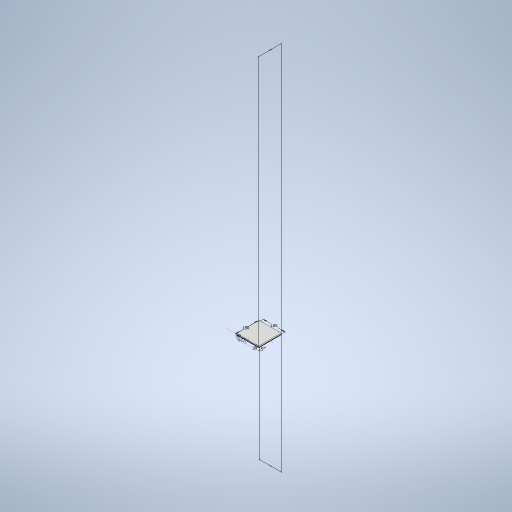
# Autodesk Inventor part: Coperchio
Saved by Autodesk Inventor 2024.2 (Build 282272000, 272)
## iProperties
Created: 2025-05-23
Part Number: Coperchio
Material: Generico
Document SubType Name: Modeling
Designer: zagom
Density: 1 g/cm^3
Appearance: Default
Author: zagom
Autodesk Inventor part; units mm, degrees
ref_plane "YZ Plane" through (0, 0, 0) normal (1, 0, 0) x (0, 1, 0)
ref_plane "XZ Plane" through (0, 0, 0) normal (0, 1, 0) x (-1, 0, 0)
ref_plane "XY Plane" through (0, 0, 0) normal (0, 0, 1) x (1, 0, 0)
sketch "Schizzo1" plane through (0, 0, 0) normal (0, 1, 0) x (-1, 0, 0)
  line L0 (-92.5, 95) -> (92.5, 95)
  line L1 (92.5, 95) -> (92.5, -95)
  line L2 (92.5, -95) -> (-92.5, -95)
  line L3 (-92.5, -95) -> (-92.5, 95)
  line L4 (-92.5, 95) -> (92.5, -95) construction
  line L5 (92.5, 95) -> (-92.5, -95) construction
  line L6 (118.5475, 95) -> (118.5475, 92.5) construction
  line L7 (103.3404, 0) -> (-125.0969, 0) construction
  line L8 (-92.5, 105.425) -> (-72.5, 105.425) construction
  line L9 (-72.5, 105.425) -> (-72.5, 79.9214) construction
  line L10 (-107.0445, 95) -> (-107.0445, 90) construction
  line L11 (-107.0445, 90) -> (178.9219, 90) construction
  line L12 (92.5, 110.0374) -> (62.5, 110.0374) construction
  line L13 (62.5, 110.0374) -> (62.5, 64.1892) construction
  line L14 (62.5, 124.2105) -> (-5, 124.2105) construction
  line L15 (-5, 124.2105) -> (-72.5, 124.2105) construction
  line L16 (-5, 124.2105) -> (-5, 64.1892) construction
  point P0 (0, 0)
  point P1 (62.5, 90)
  point P2 (-72.5, 90)
  point P3 (-5, 90)
  dimension "d0" = 185
  dimension "d1" = 190
  dimension "d39" = 20
  dimension "d40" = 5
  dimension "d41" = 30
  dimension "d57" = 67.5
  constraints: 34 end point, 7 point on line, 6 horizontal, 5 perpendicular, 2 midpoint, 2 parallel, 2 vertical
  measures "d0" distance of L1.end L2.end
  measures "d1" distance of L0.end L1.end
  measures "d39" distance of L8.start L8.end
  measures "d40" distance of L10.start L10.end
  measures "d41" distance of L12.start L12.end
  measures "d57" distance of L14.start L14.end
extrude "Estrusione1" add sketch "Schizzo1" along normal blind 10
ref_plane "Piano di lavoro1" through (-103.3404, 0, 0) normal (0, 0, 1) x (1, 0, 0)
hole "Foro5" at (-62.5, 0, 90) at (72.5, 0, 90) at (5, 0, 90) direction (0, 1, 0) diameter 3 depth 10 countersink diameter 4 countersink angle 90
mirror "Speculare4" about plane through (-103.3404, 0, 0) normal (0, 0, 1) of "Foro5"
